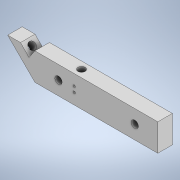
# Autodesk Inventor part: main_frame
Saved by Autodesk Inventor 2022.2 (Build 262287010, 287A)
## iProperties
Created: 2022-05-04
Part Number: main_frame
Material: Genérico
Document SubType Name: Modeling
Designer: 19710060
Density: 1 g/cm^3
Appearance: Padrão
Author: 19710060
Autodesk Inventor part; units mm, degrees
ref_plane "YZ Plane" through (0, 0, 0) normal (1, 0, 0) x (0, 1, 0)
ref_plane "XZ Plane" through (0, 0, 0) normal (0, 1, 0) x (-1, 0, 0)
ref_plane "XY Plane" through (0, 0, 0) normal (0, 0, 1) x (1, 0, 0)
sketch "Esboço1" plane through (0, 0, 0) normal (0, 0, 1) x (1, 0, 0)
  line L0 (0, 0) -> (101.5, 0)
  line L1 (0, 0) -> (-22.5, 22.5)
  line L2 (0, 0) -> (30, 0) construction
  line L3 (101.5, 0) -> (101.5, 22.5)
  line L4 (-22.5, 22.5) -> (-11.8934, 22.5)
  line L5 (-11.8934, 22.5) -> (-4.8223, 15.4289)
  line L6 (-4.8223, 15.4289) -> (0, 22.5)
  line L7 (101.5, 22.5) -> (0, 22.5)
  line L8 (-11.8934, 22.5) -> (-22.5, 22.5)
  line L9 (-22.5, 22.5) -> (-34.2669, 34.2669)
  line L10 (-4.8223, 15.4289) -> (-28.9636, 39.5702)
  dimension "d0" = 101.5
  dimension "d2" = 135
  dimension "d3" = 22.5
  dimension "d5" = 10
  dimension "d51" = 7.5
  constraints: 22 end point, 4 horizontal, 1 point on line, 1 vertical
  measures "d0" distance of L0.start L0.end
  measures "d2" angle of L2 L1
  measures "d3" distance of L0.end L3.end
  measures "d5" distance of L4.end L5.end
  measures "d51" distance between parallel lines of L9 L10
extrude "Extrusão1" add sketch "Esboço1" against normal blind 12
sketch "Esboço2" plane through (0, 0, 0) normal (0, 0, 1) x (1, 0, 0)
  line L0 (101.5, 22.5) -> (101.5, 0) projected
  line L1 (0, 0) -> (-22.5, 22.5) projected
  line L2 (0, 22.5) -> (101.5, 22.5) projected
  line L3 (101.5, 22.5) -> (82.5, 22.5)
  point P0 (82.5, 11.25)
  point P1 (19.5, 11.25)
  point P2 (32.5, 13.45)
  point P3 (32.5, 9.05)
  constraints: 2 end point, 1 point on line
hole "Furo1" at (82.5, 11.25, 0) at (19.5, 11.25, 0) direction (0, 0, -1) diameter 6 end through all
hole "Furo2" at (32.5, 13.45, 0) direction (0, 0, -1) diameter 2 depth 7
hole "Furo3" at (32.5, 9.05, 0) direction (0, 0, -1) diameter 2 end through all
sketch "Esboço3" plane through (-4.8223, 15.4289, -12) normal (0.7071068, 0.7071068, 0) x (-0.7071068, 0.7071068, 0)
  line L0 (0, 12) -> (0, 0) projected
  line L1 (0, 6) -> (5, 6)
  point P0 (-14.3198, 12)
  dimension "d34" = 5
  constraints: 2 end point, 1 horizontal, 1 midpoint
  measures "d34" distance of L1.start L1.end
hole "Furo4" at (-8.3579, 18.9645, -6) direction (-0.7071068, -0.7071068, 0) diameter 6 end through all
sketch "Esboço4" plane through (0, 22.5, 0) normal (0, 1, 0) x (1, 0, 0)
  line L0 (0, 0) -> (0, 12) projected
  line L1 (0, 12) -> (0, 6)
  line L2 (101.5, 12) -> (0, 12) projected
  line L3 (33.5, 0) -> (31.5, 0) projected
  line L4 (32.5, 0) -> (32.5, 6)
  dimension "d42" = 6
  constraints: 4 end point, 2 midpoint
  measures "d42" distance of L0.end L1.end
hole "Furo5" at (32.5, 22.5, -6) direction (0, -1, 0) diameter 2 depth 18 counterbore diameter 6 counterbore depth 6
fillet "Arredondamento1" [suppressed]
